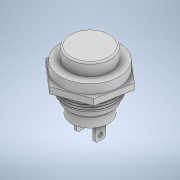
# Autodesk Inventor part: Кнопка2
Saved by Autodesk Inventor 2020 (Build 240168000, 168)
## iProperties
Created: 2020-02-08
Part Number: Кнопка2
Material: Типовые
Document SubType Name: Modeling
Designer: Andre
Density: 1 g/cm^3
Appearance: По умолчанию
Author: Andre
Autodesk Inventor part; units mm, degrees
ref_plane "YZ Plane" through (0, 0, 0) normal (1, 0, 0) x (0, 1, 0)
ref_plane "XZ Plane" through (0, 0, 0) normal (0, 1, 0) x (-1, 0, 0)
ref_plane "XY Plane" through (0, 0, 0) normal (0, 0, 1) x (1, 0, 0)
sketch "Эскиз1" plane through (0, 0, 0) normal (0, 1, 0) x (-1, 0, 0)
  circle A0 centre (0, 0) radius 6
  dimension "d0" = 12
  constraints: 1 centre point, 1 coincident
  measures "d0" diameter of A0
extrude "Выдавливание1" add sketch "Эскиз1" along normal mid plane 3
sketch "Эскиз2" plane through (0, -1.5, 0) normal (0, -1, 0) x (1, 0, 0)
  line L0 (-3.4, 1.7) -> (-2.6, 1.7)
  line L1 (-2.6, 1.7) -> (-2.6, -1.7)
  line L2 (-2.6, -1.7) -> (-3.4, -1.7)
  line L3 (-3.4, -1.7) -> (-3.4, 1.7)
  line L4 (-2.6, -1.7) -> (-3, -1.7)
  line L5 (2.6, 1.7) -> (3.4, 1.7)
  line L6 (3.4, 1.7) -> (3.4, -1.7)
  line L7 (3.4, -1.7) -> (2.6, -1.7)
  line L8 (2.6, -1.7) -> (2.6, 1.7)
  line L9 (3.4, -1.7) -> (3, -1.7)
  point P0 (0, 0)
  dimension "d5" = 0.8
  dimension "d6" = 3.4
  dimension "d9" = 0.8
  dimension "d10" = 3.4
  constraints: 20 end point, 4 parallel, 2 horizontal, 2 midpoint, 2 perpendicular
  measures "d5" distance of L1.end L2.end
  measures "d6" distance of L1.end L0.end
  measures "d9" distance of L6.end L7.end
  measures "d10" distance of L6.end L5.end
extrude "Выдавливание2" add sketch "Эскиз2" along normal blind 6
chamfer "Фаска1" distance 0.5 angle 45 4 edges at (-3, -7.5, -1.7) (3, -7.5, -1.7) (-3, -7.5, 1.7) (3, -7.5, 1.7)
sketch "Эскиз3" plane through (-3.4, -1.5, -1.7) normal (-1, 0, 0) x (0, 0, 1)
  line L0 (0.5, -6) -> (2.9, -6) projected
  line L1 (2.9, -6) -> (1.7, -6)
  line L2 (1.7, -6) -> (1.7, -4.5)
  circle A0 centre (1.7, -4.5) radius 0.75
  point P0 (1.7, 1.5)
  dimension "d20" = 1.2
  dimension "d21" = 1.5
  dimension "d22" = 1.5
  constraints: 4 end point, 1 centre point, 1 coincident, 1 midpoint, 1 perpendicular
  measures "d20" distance of L0.end L1.end
  measures "d21" distance of L1.end L2.end
  measures "d22" diameter of A0
hole "Отверстие1" at (-3.4, -6, 0) direction (1, 0, 0) diameter 1.5 end through all
sketch "Эскиз4" plane through (0, 1.5, 0) normal (0, 1, 0) x (1, 0, 0)
  circle A0 centre (0, 0) radius 7
  dimension "d31" = 14
  constraints: 1 centre point, 1 coincident
  measures "d31" diameter of A0
extrude "Выдавливание3" add sketch "Эскиз4" along normal blind 10
chamfer "Фаска2" distance 1 angle 45 1 edges at (-7, 1.5, 0)
sketch "Эскиз5" plane through (0, 11.5, 0) normal (0, 1, 0) x (1, 0, 0)
  circle A0 centre (0, 0) radius 9.5
  dimension "d37" = 19
  constraints: 1 centre point, 1 coincident
  measures "d37" diameter of A0
extrude "Выдавливание4" add sketch "Эскиз5" against normal blind 1 separate body
sketch "Эскиз6" plane through (0, 11.5, 0) normal (0, 1, 0) x (1, 0, 0)
  circle A0 centre (0, 0) radius 8
  dimension "d40" = 16
  constraints: 1 centre point, 1 coincident
  measures "d40" diameter of A0
extrude "Выдавливание5" add sketch "Эскиз6" against normal blind 7 separate body
sketch "Эскиз7" plane through (0, 11.5, 0) normal (0, 1, 0) x (1, 0, 0)
  circle A0 centre (0, 0) radius 9.5
  dimension "d45" = 19
  constraints: 1 centre point, 1 coincident
  measures "d45" diameter of A0
extrude "Выдавливание6" add sketch "Эскиз7" along normal blind 2 bodies 2
sketch "Эскиз8" plane through (0, 13.5, 0) normal (0, 1, 0) x (1, 0, 0)
  circle A0 centre (0, 0) radius 6.75
  circle A1 centre (0, 0) radius 7
  dimension "d48" = 13.5
  dimension "d52" = 14
  constraints: 2 centre point, 2 coincident
  measures "d48" diameter of A0
  measures "d52" diameter of A1
extrude "Выдавливание7" add sketch "Эскиз8" along normal blind 4 contours A0 bodies 2
thread "Резьба5" size "M16x0.75" class "4g6g" standard "ANSI Metric M Profile" full length
fillet "Сопряжение1" radius 0.5 1 edges at (-6.75, 17.5, 0)
sketch "Эскиз9" plane through (0, 13.5, 0) normal (0, 1, 0) x (1, 0, 0)
  point P0 (0, 0)
sketch "Эскиз10" plane through (0, 10.5, 0) normal (0, -1, 0) x (1, 0, 0)
  point P0 (0, 0)
sketch "Эскиз11" plane through (0, 10.5, 0) normal (0, -1, 0) x (1, 0, 0)
  point P0 (0, 0)
sketch "Эскиз12" plane through (0, 10.5, 0) normal (0, -1, 0) x (1, 0, 0)
  line L0 (-8.586, -7.3361) -> (-10.6462, 3.7676)
  line L1 (-10.6462, 3.7676) -> (-2.0603, 11.1037)
  line L2 (-2.0603, 11.1037) -> (8.586, 7.3361)
  line L3 (8.586, 7.3361) -> (10.6462, -3.7676)
  line L4 (10.6462, -3.7676) -> (2.0603, -11.1037)
  line L5 (2.0603, -11.1037) -> (-8.586, -7.3361)
  point P0 (0, 0)
  point P1 (0, 0)
  constraints: 12 end point, 1 coincident, 13 other
extrude "Выдавливание8" add sketch "Эскиз12" along normal blind 2.2 bodies 2
fillet "Сопряжение2" radius 0.2 6 edges at (9.6161, 8.3, 1.7842) (6.3532, 8.3, -7.4357) (-3.2628, 8.3, -9.2199) (-9.6161, 8.3, -1.7842) (3.2628, 8.3, 9.2199) (-6.3532, 8.3, 7.4357)
sketch "Эскиз14" plane through (0, 4.5, 0) normal (-1, 0, 0) x (0, 0, 1)
  line L0 (8, 0) -> (8, 7)
  line L1 (8, 7) -> (7.4439, 7)
  line L2 (7.4439, 7) -> (7.4439, 0)
  line L3 (7.4439, 0) -> (8, 0)
  line L4 (0, -17) -> (0, 18) projected
  constraints: 8 end point
revolve "Вращение1" cut sketch "Эскиз14" angle 360 about axis through (0, 4.5, 0) along (0, 1, 0) bodies 1
sketch "Эскиз15" plane through (0, 4.5, 0) normal (-1, 0, 0) x (0, 0, 1)
  line L0 (8, 0) -> (8, 7)
  line L1 (8, 7) -> (7.4439, 7)
  line L2 (7.4439, 7) -> (7.4439, 0)
  line L3 (7.4439, 0) -> (8, 0)
  line L4 (0, -17) -> (0, 18) projected
  constraints: 8 end point
revolve "Вращение2" add sketch "Эскиз15" angle 360 about axis through (0, 4.5, 0) along (0, 1, 0) separate body
sketch "Эскиз13" plane through (0, 4.5, 0) normal (1, 0, 0) x (0, 1, 0)
  line L0 (-0.4376, -7.482) -> (-0.3751, -7.482) construction
  line L1 (0.0624, -7.9622) -> (-0.0001, -8.0823) construction
  line L2 (-0.7501, -8.0823) -> (-0.8126, -7.9622) construction
  line L3 (-0.3126, -7.482) -> (-0.3751, -7.3619) construction
  line L4 (-0.3751, -7.3619) -> (-0.4376, -7.482) construction
  line L5 (-0.7501, -8.0823) -> (-0.6876, -7.9622) construction
  line L6 (-0.3126, -7.482) -> (-0.0626, -7.9622)
  line L7 (-0.8126, -7.9622) -> (-0.6876, -7.9622) construction
  arc A0 (-0.8126, -7.9622) -> (-0.7501, -8.0002) centre (-0.7501, -7.9297) ccw construction
  line L8 (0.0624, -7.9622) -> (-0.0626, -7.9622) construction
  line L9 (-0.7501, -8.0823) -> (-0.7501, -7.9622) construction
  line L10 (-0.0001, -8.0823) -> (-0.0001, -7.9622) construction
  line L11 (-0.3751, -7.3619) -> (-0.3751, -7.4441) construction
  line L12 (-0.7501, -8.0002) -> (-0.0001, -8.0002)
  arc A1 (-0.7501, -8.0002) -> (-0.6876, -7.9622) centre (-0.7501, -7.9297) ccw
  line L13 (-0.0626, -7.9622) -> (-0.0001, -8.0823) construction
  line L14 (-0.6876, -7.9622) -> (-0.4376, -7.482)
  line L15 (-0.0001, -0.0002) -> (-0.0001, 0.0177)
  line L16 (-0.0001, 0.0177) -> (-0.0001, -0.0002)
  line L17 (-0.0001, -0.0002) -> (0.0334, -0.0002)
  arc A2 (-0.0626, -7.9622) -> (-0.0001, -8.0002) centre (-0.0001, -7.9297) ccw
  arc A3 (-0.0001, -8.0002) -> (0.0624, -7.9622) centre (-0.0001, -7.9297) ccw construction
  arc A4 (-0.3751, -7.4441) -> (-0.4376, -7.482) centre (-0.3751, -7.5145) ccw
  arc A5 (-0.3126, -7.482) -> (-0.3751, -7.4441) centre (-0.3751, -7.5145) ccw
  line L18 (-0.3751, -7.4441) -> (-0.3751, -7.482) construction
  line L19 (-0.3751, -7.482) -> (-0.3126, -7.482) construction
  dimension "d65" = 55
  dimension "d66" = 0.1201
  dimension "d67" = 0.1201
  dimension "Эскиз13_ThreadOffset" = 0
  dimension "Эскиз13_MajorRadius" = 8
  dimension "d70" = 0.75
  dimension "Эскиз13_MinorRadius" = 7.4439
  constraints: 40 end point, 12 point on circle, 10 parallel, 8 tangent, 6 centre point, 6 collinear, 2 midpoint, 2 point on line, 1 horizontal, 1 perpendicular, 3 other
  measures "d65" angle of L6 L14
  measures "d66" distance of L3.end L0.end
  measures "d67" distance of L1.end L10.end
  measures "Эскиз13_ThreadOffset" distance between parallel lines of L15 L10
  measures "Эскиз13_MajorRadius" distance from line of L12 L15.start
  measures "d70" distance from line of L1.end L9
  measures "Эскиз13_MinorRadius" distance edge to line of A5 L17
coil "Пружина1" sketch "Эскиз13" operation cut axis through (0, 4.5, 0) along (0, 1, 0) pitch 0.7508 turns 11.322011 hand right bodies 4
equation "\"d65\" = d72"
equation "\"d66\" = 0.160083 * Эскиз13_Pitch"
equation "\"d67\" = 0.160083 * Эскиз13_Pitch"
equation "\"d70\" = Эскиз13_Pitch"
equation "\"d72\" = 55deg"
equation "\"Эскиз13_Pitch\" = 0.75"
